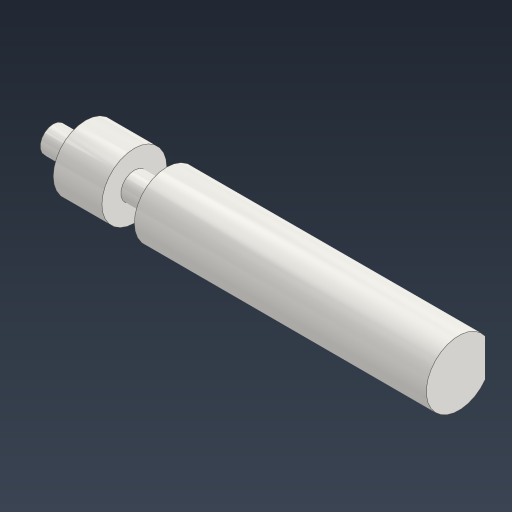
# Autodesk Inventor part: Shaft
Saved by Autodesk Inventor 2023 (Build 270158000, 158)
## iProperties
Created: 2025-04-27
Part Number: Shaft
Material: Steel
Document SubType Name: Modeling
Designer: szymo
Density: 1 g/cm^3
Appearance: Steel
Author: szymo
Length: 37.500 mm
Autodesk Inventor part; units mm, degrees
ref_plane "Start Plane" through (0, 0, 0) normal (1, 0, 0) x (0, 1, 0)
ref_plane "XZ Plane" through (0, 0, 0) normal (0, 1, 0) x (-1, 0, 0)
ref_plane "XY Plane" through (0, 0, 0) normal (0, 0, 1) x (1, 0, 0)
sketch "Main Sketch" plane through (0, 0, 0) normal (0, 0, 1) x (1, 0, 0)
  line L0 (0, 0) -> (37.5, 0)
  line L1 (0, 0) -> (0, 1.205)
  line L2 (0, 1.205) -> (3, 1.205)
  line L3 (3, 1.205) -> (3, 3)
  line L4 (7.5, 3) -> (7.5, 1.25)
  line L5 (3, 3) -> (7.5, 3)
  line L6 (7.5, 1.25) -> (10.5, 1.25)
  line L7 (10.5, 1.25) -> (10.5, 3)
  line L8 (37.5, 3) -> (37.5, 0)
  line L9 (10.5, 3) -> (37.5, 3)
  dimension "d3" = 2.41
  dimension "d4" = 6
  dimension "d5" = 2.5
  dimension "d6" = 6
  constraints: 20 end point, 6 horizontal, 5 vertical
  measures "d3" diameter of L2 L0
  measures "d4" diameter of L5 L0
  measures "d5" diameter of L6 L0
  measures "d6" diameter of L9 L0
revolve "Revolution1" add sketch "Main Sketch" angle 360 about axis through (0, 0, 0) along (1, 0, 0)
sketch "Sketch3" plane through (37.5, 0, 0) normal (1, 0, 0) x (0, 0, -1)
  circle A0 centre (0, 0) radius 3 projected
  circle A1 centre (0, 0) radius 3 projected
  line L0 (2.45, 1.7313) -> (2.45, -1.7313)
  dimension "d8" = 5.45
  constraints: 2 end point, 2 point on circle, 1 vertical
extrude "Extrusion1" cut sketch "Sketch3" against normal blind 11.5 contours A0 L0 picked at (2.5504, -0.3987)
equation "\"Length\" = 37.5"
body "Solid1"
